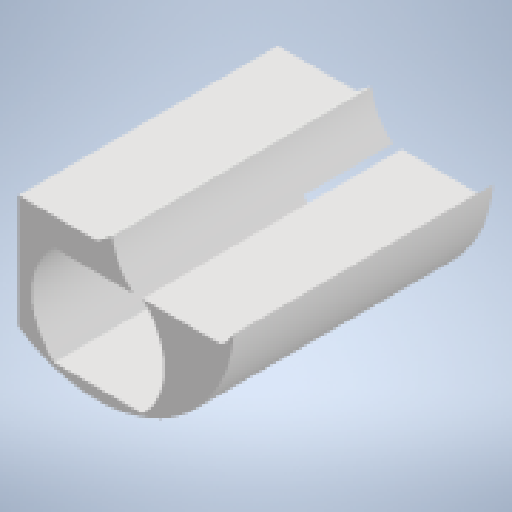
# Autodesk Inventor part: ROTATE
Saved by Autodesk Inventor 2023.2 (Build 272271030, 271C)
## iProperties
Created: 2023-06-22
Part Number: ROTATE
Material: Generic
Document SubType Name: Modeling
Designer: kao91
Density: 1 g/cm^3
Appearance: Default
Author: kao91
Autodesk Inventor part; units mm, degrees
ref_plane "YZ Plane" through (0, 0, 0) normal (1, 0, 0) x (0, 1, 0)
ref_plane "XZ Plane" through (0, 0, 0) normal (0, 1, 0) x (-1, 0, 0)
ref_plane "Work Plane1" through (-51.0014, -51.0767, 47.0039) normal (0, 0, -1) x (0, 1, 0)
sketch "Sketch1" plane through (0, 0, 0) normal (0, 0, 1) x (1, 0, 0)
  arc A0 (-51.0008, -8.0945) -> (-16.665, 27.298) centre (-36.8015, 12.4817) ccw
  line L0 (15.6539, 51.0767) -> (-36.8027, 12.4817) projected
  line L1 (-36.8027, 12.4817) -> (-51.0008, 12.4817) projected
  line L2 (-51.0008, 12.4817) -> (-51.0008, -51.0767) projected
  line L3 (-15.3897, 25.4817) -> (-29.0068, 25.4817) projected
  line L4 (-14.1984, 25.4817) -> (-15.3897, 25.4817) projected
  ellipse E0 centre (-22.3234, 16.4817) end of major axis (-22.3234, 28.6067) minor radius 12.125 (-14.1984, 7.4817) -> (-14.1984, 25.4817) ccw projected
  line L5 (-15.3897, 7.4817) -> (-14.1984, 7.4817) projected
  line L6 (-29.0068, 7.4817) -> (-15.3897, 7.4817) projected
  line L7 (-30.1984, 7.4817) -> (-29.0068, 7.4817) projected
  ellipse E1 centre (-22.0734, 16.4817) end of major axis (-22.0734, 4.3567) minor radius 12.125 (-30.1984, 25.4817) -> (-30.1984, 7.4817) ccw projected
  line L8 (-44.552, -10.5183) -> (-37.9322, -10.5183) projected
  line L9 (-37.9322, -10.5183) -> (-35.1718, -10.5183) projected
  line L10 (-35.1718, -10.5183) -> (-28.552, -10.5183) projected
  arc A1 (-28.552, -10.5183) -> (-24.6451, -3.0183) centre (-36.677, -1.5183) ccw projected
  arc A2 (-28.552, -10.5183) -> (-28.552, 7.4817) centre (-36.677, -1.5183) ccw projected
  line L11 (-35.2148, 7.4817) -> (-28.552, 7.4817) projected
  line L12 (-35.2148, 7.4817) -> (-37.8892, 7.4817) projected
  line L13 (-44.552, 7.4817) -> (-37.8892, 7.4817) projected
  arc A3 (-44.552, 7.4817) -> (-46.3273, 5.4817) centre (-36.427, -1.5183) ccw projected
  ellipse E2 centre (-36.4279, -1.5183) end of major axis (-36.4279, -13.1433) minor radius 11.625 (-44.3583, 6.9817) -> (-44.3583, -10.0183) ccw projected
  arc A4 (-46.3273, 5.4817) -> (-48.4589, -0.0183) centre (-36.427, -1.5183) ccw projected
  arc A5 (-44.552, 7.4817) -> (-44.552, -10.5183) centre (-36.427, -1.5183) ccw projected
  point P0 (0, 0)
  point P1 (-11.8976, 10.2915)
  point P2 (-34.0379, 14.5159)
  point P3 (-15.4473, 25.4817)
  point P4 (-19.1337, 25.4817)
  point P5 (-16.6653, 27.2981)
  point P6 (-51.0008, -8.0945)
  dimension "d0" = 50
  constraints: 2 point on circle, 2 point on line, 1 centre point, 3 other
  measures "d0" diameter of A0
extrude "Extrusion1" add sketch "Sketch1" along normal up to surface (47.0015 mm away) contours L2 L1 L0 E1 L11 L12 L13 A3 A4 A5 L8 L9 L10 A1 A2 L6 L5 E0 A0
body "Solid1"
